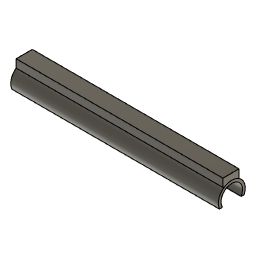
External1 (Autodesk Fusion 360 design; units mm, degrees)
Autodesk Fusion 360 part; units mm, degrees
derive "DerivedContext1" from "Ensamble dron BPI v12"
sketch "Sketch1" plane through (0, 0, 0) normal (0, 0, 1) x (1, 0, 0)
  line L0 (-25.5859, -33.0067, 81.57) -> (51.3864, -33.0067, 81.57)
  line L1 (-25.434, -35.9918) -> (51.2526, -35.9918)
  line L2 (12.994, -32.9965) -> (51.4685, -33.0066)
  line L3 (-25.4324, -29.9808) -> (51.2542, -30.0213)
  line L4 (51.2542, -30.0213) -> (51.2526, -35.9918)
  line L5 (-25.4324, -29.9808) -> (-25.434, -35.9918)
  constraint symmetric L1.start L2 L3.start
  constraint symmetric L1.end L2 L3.end
extrude "Extrude1" add sketch "Sketch1" along normal blind 3 makes body 1
sketch "Sketch2" plane through (-25.4244, 0.0067, 0) normal (-1, 0.000264, 0) x (-0.000264, -1, 0)
  line L0 (29.9875, 0) -> (35.9986, 0)
  line L1 (35.9986, 0) -> (35.9986, 3)
  line L2 (35.9986, 3) -> (29.9875, 3)
  line L3 (29.9875, 3) -> (29.9875, 0)
  line L4 (32.993, 0) -> (32.993, -4)
  arc A0 (37.5929, -5.9599) -> (28.3931, -5.9599) centre (32.993, -4) ccw
  arc A1 (36.48, -5.9599) -> (29.506, -5.9599) centre (32.993, -4) ccw
  line L5 (37.5929, -5.9599) -> (36.48, -5.9599)
  line L6 (29.506, -5.9599) -> (28.3931, -5.9599)
  dimension "d3" = 4
  dimension "d8" = 8
  dimension "d9" = 10
  constraint midpoint L0 L4.start
  constraint perpendicular L0 L4
  constraint coincident L4.end A0.centre
  constraint concentric A0 A1
  constraint parallel L0 L5
  constraint coincident A1.end L5
  constraint collinear L5 L6
  measures "d3" distance of L4.start L4.end
  measures "d8" diameter of A1
  measures "d9" diameter of A0
extrude "Extrude2" add sketch "Sketch2" against normal blind 77 separate body contours L0 A0 | L0 A0 A1 L6 | L0 A0 A1 L5 makes body 2
